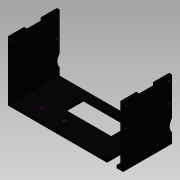
# Autodesk Inventor part: Kepala Tengah 2
Saved by Autodesk Inventor 2015 SP1 (Build 190203100, 203)
## iProperties
Created: 2015-02-05
Part Number: Kepala Tengah 2
Material: Generic
Document SubType Name: Modeling
Designer: Rafi Kurnia Putra
Density: 1 g/cm^3
Appearance: Anodized - Black
Mass: 42.602 g
Surface Area: 265.911 cm^2
Volume: 42.602 cm^3
Author: Rafi Kurnia Putra
Autodesk Inventor part; units mm, degrees
ref_plane "YZ Plane" through (0, 0, 0) normal (1, 0, 0) x (0, 1, 0)
ref_plane "XZ Plane" through (0, 0, 0) normal (0, 1, 0) x (-1, 0, 0)
sketch "Sketch1" plane through (0, 0, 0) normal (0, 1, 0) x (-1, 0, 0)
  line L0 (60.406, 25.6071) -> (-60.406, 25.6071)
  line L1 (-60.406, 25.6071) -> (-60.406, -25.6071)
  line L2 (-60.406, -25.6071) -> (60.406, -25.6071)
  line L3 (60.406, -25.6071) -> (60.406, 25.6071)
  line L4 (60.406, 25.6071) -> (-60.406, -25.6071) construction
  line L5 (-60.406, 25.6071) -> (60.406, -25.6071) construction
  line L6 (-57.406, 25.6071) -> (-57.406, -25.6071)
  line L7 (57.406, -25.6071) -> (57.406, 25.6071)
  line L8 (57.406, 23.5058) -> (55.4493, 23.5058)
  line L9 (-55.4493, 23.5058) -> (-57.406, 23.5058)
  line L10 (-57.406, -33.4947) -> (-79.0126, -33.4947)
  line L11 (79.0126, -33.4947) -> (57.406, -33.4947)
  point P0 (0, 0)
  dimension "d0" = 120.812
  dimension "d1" = 51.2141
  dimension "d8" = 3
  dimension "d9" = 3
  dimension "d10" = 114.812
  constraints: 24 end point, 12 point on line, 7 parallel, 3 perpendicular, 2 midpoint, 1 horizontal
  measures "d0" distance of L2.end L1.end
  measures "d1" distance of L1.end L0.end
  measures "d8" distance between parallel lines of L7 L3
  measures "d9" distance between parallel lines of L6 L1
  measures "d10" distance between parallel lines of L7 L6
extrude "Extrusion1" add sketch "Sketch1" along normal blind 3
extrude "Extrusion2" add sketch "Sketch1" along normal blind 63 contours L3 L2 L7 L0 | L6 L2 L1 L0
ref_plane "Work Plane2" through (0, 0, -18.4174) normal (0, 0, 1) x (1, 0, 0)
sketch "Sketch2" plane through (0, 0, 0) normal (0, -1, 0) x (1, 0, 0)
  circle A0 centre (-50.5968, 0.5202) radius 1.75 projected
  circle A1 centre (-28.0003, -13.4843) radius 1.75 projected
  circle A2 centre (50.5962, 0.5202) radius 1.75 projected
  circle A3 centre (27.9997, -13.4843) radius 1.75 projected
  circle A4 centre (27.9997, -13.4843) radius 1.75
  circle A5 centre (50.5962, 0.5202) radius 1.75
  circle A6 centre (-28.0003, -13.4843) radius 1.75
  circle A7 centre (-50.5968, 0.5202) radius 1.75
  point P0 (0, 0)
  dimension "d12" = 3.5
  dimension "d13" = 3.5
  dimension "d14" = 3.5
  dimension "d15" = 3.5
  constraints: 4 centre point, 4 coincident
  measures "d12" diameter of A4
  measures "d13" diameter of A5
  measures "d14" diameter of A6
  measures "d15" diameter of A7
extrude "Extrusion3" cut sketch "Sketch2" against normal up to next
sketch "Sketch4" plane through (0, 63, 0) normal (0, 1, 0) x (1, 0, 0)
  line L0 (-60.406, -8.75) -> (-56.906, -8.75)
  line L1 (-56.906, -8.75) -> (-56.906, 8.75)
  line L2 (-56.906, 8.75) -> (-60.406, 8.75)
  line L3 (-60.406, -8.75) -> (-60.406, 8.75)
  line L4 (0, 0) -> (0, 8.75)
  line L5 (60.406, -8.75) -> (56.906, -8.75)
  line L6 (56.906, -8.75) -> (56.906, 8.75)
  line L7 (56.906, 8.75) -> (60.406, 8.75)
  line L8 (60.406, -8.75) -> (60.406, 8.75)
  point P0 (-60.406, 0)
  point P1 (60.406, 0)
  dimension "d18" = 17.5
  constraints: 18 end point, 5 symmetric about line, 2 vertical, 1 horizontal, 1 parallel, 1 perpendicular
  measures "d18" distance of L1.end L0.end
extrude "Extrusion4" cut sketch "Sketch4" against normal blind 3
sketch "Sketch6" plane through (0, 0, 0) normal (0, -1, 0) x (1, 0, 0)
  circle A0 centre (-32.4423, 8.2996) radius 1.5 projected
  circle A1 centre (32.4417, 8.2996) radius 1.5 projected
  point P0 (0, 0)
extrude "Extrusion5" cut sketch "Sketch6" against normal up to next
sketch "Sketch9" plane through (60.406, 0, 25.6071) normal (1, 0, 0) x (0, 0, -1)
  circle A0 centre (3, 59.0338) radius 1 projected
  circle A1 centre (3, 38.0338) radius 1 projected
  circle A2 centre (48.2141, 59.0338) radius 1 projected
  circle A3 centre (48.2141, 38.0338) radius 1 projected
  point P0 (25.6071, 0)
extrude "Extrusion7" cut sketch "Sketch9" against normal blind 200
sketch "Sketch10" plane through (0, 0, 0) normal (0, -1, 0) x (1, 0, 0)
  circle A0 centre (-28.0003, -13.4843) radius 1.75 projected
  circle A1 centre (27.9997, -13.4843) radius 1.75 projected
  line L0 (53.5962, 73.5112) -> (-53.5968, 73.5112)
  line L1 (-24.5003, -13.4843) -> (24.4997, -13.4843)
  line L2 (24.4997, 73.5112) -> (-24.5003, 73.5112)
  line L3 (-24.5003, -13.4843) -> (-24.5003, -2.4798)
  line L4 (-24.5003, -13.4843) -> (-13.4958, -13.4843) construction
  line L5 (-24.5003, -2.4798) -> (24.4997, -2.4798)
  line L6 (24.4997, -13.4843) -> (24.4997, -2.4798)
  point P0 (0, 0)
  dimension "d39" = 90
  constraints: 14 end point, 2 horizontal, 2 perpendicular, 1 parallel, 1 point on line
  measures "d39" angle of L4 L3
extrude "Extrusion8" cut sketch "Sketch10" against normal up to next contours L3 L5 L6 L1
sketch "Sketch11" plane through (0, 0, 0) normal (0, -1, 0) x (1, 0, 0)
  circle A0 centre (-38.0003, 13.0422) radius 1.75
  circle A1 centre (-14.0003, 13.0422) radius 1.75
  line L0 (-36.0003, -4.4688) -> (-36.0003, 50.5312) projected
  line L1 (-16.0003, 50.5312) -> (-16.0003, -4.4688) projected
  line L2 (-34.6078, 15.0422) -> (34.6072, 15.0422) projected
  point P0 (0, 0)
  dimension "d31" = 3.5
  dimension "d32" = 3.5
  dimension "d33" = 2
  dimension "d34" = 2
  dimension "d37" = 2
  dimension "d38" = 2
  constraints: 2 centre point
  measures "d31" diameter of A0
  measures "d32" diameter of A1
  measures "d33" distance from line of A0.centre L0
  measures "d34" distance from line of L1 A1.centre
  measures "d37" distance from line of L2 A0.centre
  measures "d38" distance from line of L2 A1.centre
extrude "Extrusion9" cut sketch "Sketch11" against normal up to next
sketch "Sketch15" plane through (-60.406, 0, -25.6071) normal (-1, 0, 0) x (0, 0, 1)
  circle A0 centre (-6.7939, 16.9) radius 9.2 projected
  point P0 (25.6071, 0)
extrude "Extrusion11" cut sketch "Sketch15" against normal through all
sketch "Sketch16" plane through (0, 0, 0) normal (0, -1, 0) x (1, 0, 0)
  line L0 (45.6757, 24.585) -> (45.6757, 11.915) projected
  line L1 (51.4357, 11.915) -> (51.4357, 24.585) projected
  line L2 (45.6757, 11.915) -> (51.4357, 11.915) projected
  line L3 (51.4357, 24.585) -> (45.6757, 24.585) projected
  line L4 (43.5557, 27) -> (53.5557, 27)
  line L5 (53.5557, 27) -> (53.5557, 9.5)
  line L6 (53.5557, 9.5) -> (43.5557, 9.5)
  line L7 (43.5557, 9.5) -> (43.5557, 27)
  line L8 (43.5557, 27) -> (53.5557, 9.5) construction
  line L9 (53.5557, 27) -> (43.5557, 9.5) construction
  point P0 (0, 0)
  point P1 (48.5557, 18.25)
  dimension "d49" = 10
  dimension "d50" = 17.5
  constraints: 12 end point, 2 midpoint, 2 parallel, 1 horizontal, 1 perpendicular
  measures "d49" distance of L5.end L6.end
  measures "d50" distance of L4.end L5.end
extrude "Extrusion12" cut sketch "Sketch16" against normal up to next contours L3 L1 L2 L0 | L4 L5 L6 L7
sketch "Sketch17" plane through (0, 3, 0) normal (0, 1, 0) x (1, 0, 0)
  circle A0 centre (-28.0003, 13.4843) radius 1.75 projected
  circle A1 centre (27.9997, 13.4843) radius 1.75 projected
  circle A2 centre (-28.0003, 7.4843) radius 1.75
  circle A3 centre (27.9997, 7.4843) radius 1.75
  line L0 (-24.5003, 13.4843) -> (24.4997, 13.4843) projected
  line L1 (-24.5003, 2.4798) -> (-24.5003, 13.4843) projected
  circle A4 centre (-50.5968, -0.5202) radius 1.75 projected
  circle A5 centre (50.5962, -0.5202) radius 1.75 projected
  line L2 (-24.5003, -2.2702) -> (24.4997, -2.2702)
  line L3 (24.4997, -2.2702) -> (24.4997, 17.7298)
  line L4 (24.4997, 17.7298) -> (-24.5003, 17.7298)
  line L5 (-24.5003, 17.7298) -> (-24.5003, -2.2702)
  point P0 (0, 0)
  dimension "d53" = 3.5
  dimension "d54" = 6
  dimension "d55" = 6
  dimension "d56" = 20
  constraints: 8 end point, 2 centre point, 2 parallel, 1 horizontal, 1 perpendicular
  measures "d53" diameter of A3
  measures "d54" distance of A2.centre A0.centre
  measures "d55" distance of A3.centre A1.centre
  measures "d56" distance of L3.end L2.end
sketch "Sketch18" plane through (-60.406, 0, -25.6071) normal (-1, 0, 0) x (0, 0, 1)
  circle A0 centre (5, 31.008) radius 1
  line L0 (0, 0) -> (51.2141, 0) projected
  line L1 (0, 23.1035) -> (0, 63) projected
  circle A1 centre (5.7141, 5.5) radius 1
  line L2 (0, 0) -> (0, 10.6965) projected
  point P0 (25.6071, 0)
  dimension "d59" = 5
  dimension "d60" = 2
  dimension "d61" = 5.5
  dimension "d62" = 5.7141
  constraints: 2 centre point
  measures "d59" distance from line of A0.centre L1
  measures "d60" diameter of A1
  measures "d61" distance from line of L0 A1.centre
  measures "d62" distance from line of A1.centre L2
extrude "Extrusion13" cut sketch "Sketch18" against normal through all
extrude "Extrusion14" cut sketch "Sketch17" against normal through all contours A2 | A3 | L5 L4 L3 L0 | L0 L3 L2 L5 L1
equation "\"d55\" = d54"
body "Solid1"
